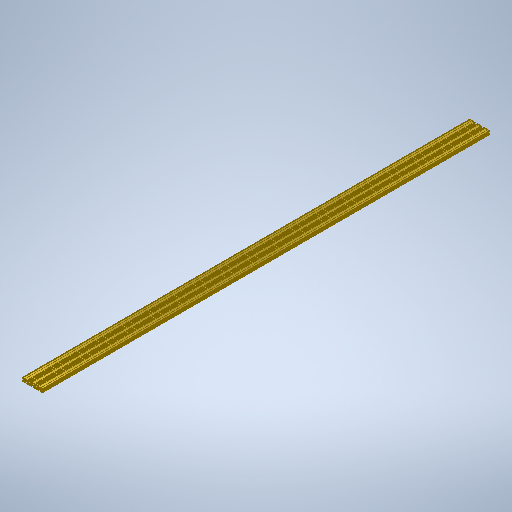
# Autodesk Inventor part: Perfil 15×90 7 rasgos_AST01509007
Saved by Autodesk Inventor 2025.2 (Build 292293000, 293)
## iProperties
Created: 2025-04-03
Part Number: Perfil 15×90 7 rasgos_AST01509007
Material: Ouro
Document SubType Name: Modeling
Designer: Gustavo Sousa
Density: 19.3 g/cm^3
Appearance: Metal quente 2400F
Author: Gustavo Sousa
Autodesk Inventor part; units mm, degrees
ref_plane "YZ Plane" through (0, 0, 0) normal (1, 0, 0) x (0, 1, 0)
ref_plane "XZ Plane" through (0, 0, 0) normal (0, 1, 0) x (-1, 0, 0)
ref_plane "XY Plane" through (0, 0, 0) normal (0, 0, 1) x (1, 0, 0)
sketch "Esboço1" plane through (0, 0, 0) normal (0, 0, 1) x (1, 0, 0)
  line L0 (-45, 7.5) -> (45, 7.5) construction
  line L1 (-45, 7.5) -> (-45, -7.5) construction
  line L2 (-39.5, 3.1) -> (-39.5, -3.1) construction
  line L3 (-45, 3.1) -> (-45, -3.1) construction
  line L4 (-45, 7.5) -> (-45, 3.1) construction
  line L5 (-45, 3.1) -> (-43.5, 3.1) construction
  line L6 (-43.5, 3.1) -> (-43.5, 6.1) construction
  line L7 (-43.5, 6.1) -> (-39.5, 3.1) construction
  line L8 (-45, -3.1) -> (-45, -7.5) construction
  line L9 (-45, -3.1) -> (-43.5, -3.1) construction
  line L10 (-43.5, -3.1) -> (-43.5, -6.1) construction
  line L11 (-43.5, -6.1) -> (-39.5, -3.1) construction
  line L12 (-45, -7.5) -> (45, -7.5) construction
  arc A0 (-44.5, 7.5) -> (-45, 7) centre (-44.5, 7) ccw
  line L13 (-45, 7) -> (-45, 3.1) construction
  line L14 (-34.1, -7.5) -> (-25.9, -7.5) construction
  line L15 (-19.1, 7.5) -> (-10.9, 7.5) construction
  line L16 (-34.1, -7.5) -> (-34.1, -5.3) construction
  line L17 (-25.9, -5.3) -> (-25.9, -7.5) construction
  line L18 (-19.1, 7.5) -> (-19.1, 5.3) construction
  line L19 (-10.9, 7.5) -> (-10.9, 5.3) construction
  line L20 (-25.9, -5.3) -> (-22.7, -5.3) construction
  line L21 (-34.1, -5.3) -> (-37.3, -5.3) construction
  line L22 (-34.1, 0.3735) -> (-25.9, 0.3735) construction
  line L23 (-19.1, -0.3735) -> (-10.9, -0.3735) construction
  line L24 (-25.9, 0.3735) -> (-22.7, -1.1206) construction
  line L25 (-22.3, 1.1206) -> (-19.1, -0.3735) construction
  line L26 (-22.7, -1.1206) -> (-22.7, -5.3) construction
  line L27 (-37.3, -1.1206) -> (-37.3, -5.3) construction
  line L28 (-37.3, -1.1206) -> (-34.1, 0.3735) construction
  line L29 (-19.1, 5.3) -> (-22.3, 5.3) construction
  line L30 (-22.3, 5.3) -> (-22.3, 1.1206) construction
  line L31 (-10.9, 5.3) -> (-7.7, 5.3) construction
  line L32 (-7.7, 5.3) -> (-7.7, 1.1206) construction
  line L33 (-7.7, 1.1206) -> (-10.9, -0.3735) construction
  line L34 (-45, 3.1) -> (-44.5, 3.1) construction
  line L35 (-44.5, 3.1) -> (-44.5, 3.6)
  line L36 (-44.5, 3.6) -> (-45, 3.6)
  line L37 (-45, 3.6) -> (-45, 3.1) construction
  line L38 (-45, 7) -> (-45, 3.6)
  line L39 (-44.5, 3.1) -> (-43.5, 3.1)
  arc A1 (-39.5, 2.85) -> (-39.7, 3.25) centre (-40, 2.85) ccw
  arc A2 (-42.7, 5.5) -> (-43.5, 5.1) centre (-43, 5.1) ccw
  arc A3 (-39.7, -3.25) -> (-39.5, -2.85) centre (-40, -2.85) ccw
  arc A4 (-43.5, -5.1) -> (-42.7, -5.5) centre (-43, -5.1) ccw
  line L40 (-43.5, 5.1) -> (-43.5, 3.1)
  line L41 (-42.7, 5.5) -> (-39.7, 3.25)
  line L42 (-39.5, 2.85) -> (-39.5, -2.85)
  line L43 (-42.7, -5.5) -> (-39.7, -3.25)
  line L44 (-43.5, -5.1) -> (-43.5, -3.1)
  line L45 (-45, -3.1) -> (-44.5, -3.1) construction
  line L46 (-44.5, -3.1) -> (-44.5, -3.6)
  line L47 (-44.5, -3.6) -> (-45, -3.6)
  line L48 (-45, -3.6) -> (-45, -3.1) construction
  line L49 (-44.5, -3.1) -> (-43.5, -3.1)
  arc A5 (-45, -7) -> (-44.5, -7.5) centre (-44.5, -7) ccw
  line L50 (-45, -3.6) -> (-45, -7)
  line L51 (-34.1, -7.5) -> (-34.6, -7.5) construction
  line L52 (-34.6, -7.5) -> (-34.6, -7)
  line L53 (-34.6, -7) -> (-34.1, -7)
  line L54 (-34.1, -7) -> (-34.1, -7.5) construction
  line L55 (-44.5, -7.5) -> (-34.6, -7.5)
  line L56 (-34.1, -7) -> (-34.1, -5.3)
  arc A6 (-37.3, -4.8) -> (-36.8, -5.3) centre (-36.8, -4.8) ccw
  arc A7 (-37.0115, -0.9859) -> (-37.3, -1.439) centre (-36.8, -1.439) ccw
  arc A8 (-33.989, 0.3735) -> (-34.2006, 0.3266) centre (-33.989, -0.1265) ccw
  arc A9 (-25.7994, 0.3266) -> (-26.011, 0.3735) centre (-26.011, -0.1265) ccw
  arc A10 (-22.7, -1.439) -> (-22.9885, -0.9859) centre (-23.2, -1.439) ccw
  arc A11 (-23.2, -5.3) -> (-22.7, -4.8) centre (-23.2, -4.8) ccw
  line L57 (-34.1, -5.3) -> (-36.8, -5.3)
  line L58 (-37.3, -4.8) -> (-37.3, -1.439)
  line L59 (-37.0115, -0.9859) -> (-34.2006, 0.3266)
  line L60 (-33.989, 0.3735) -> (-26.011, 0.3735)
  line L61 (-25.7994, 0.3266) -> (-22.9885, -0.9859)
  line L62 (-22.7, -1.439) -> (-22.7, -4.8)
  line L63 (-23.2, -5.3) -> (-25.9, -5.3)
  line L64 (-25.9, -7.5) -> (-25.4, -7.5) construction
  line L65 (-25.4, -7.5) -> (-25.4, -7)
  line L66 (-25.4, -7) -> (-25.9, -7)
  line L67 (-25.9, -7) -> (-25.9, -7.5) construction
  line L68 (-25.9, -5.3) -> (-25.9, -7)
  line L69 (-4.1, -7.5) -> (4.1, -7.5) construction
  line L70 (-4.1, -5.3) -> (-4.1, -7.5) construction
  line L71 (-7.3, -5.3) -> (-4.1, -5.3) construction
  line L72 (-7.3, -5.3) -> (-7.3, -1.1206) construction
  line L73 (-4.1, 0.3735) -> (4.1, 0.3735) construction
  line L74 (-7.3, -1.1206) -> (-4.1, 0.3735) construction
  line L75 (-4.1, -7.5) -> (-4.6, -7.5) construction
  line L76 (-4.6, -7.5) -> (-4.6, -7)
  line L77 (-4.6, -7) -> (-4.1, -7)
  line L78 (-4.1, -7) -> (-4.1, -7.5) construction
  line L79 (-4.1, -5.3) -> (-4.1, -7)
  arc A12 (-7.3, -4.8) -> (-6.8, -5.3) centre (-6.8, -4.8) ccw
  arc A13 (-7.0115, -0.9859) -> (-7.3, -1.439) centre (-6.8, -1.439) ccw
  arc A14 (-3.989, 0.3735) -> (-4.2006, 0.3266) centre (-3.989, -0.1265) ccw
  line L80 (-6.8, -5.3) -> (-4.1, -5.3)
  line L81 (-7.3, -4.8) -> (-7.3, -1.439)
  line L82 (-7.0115, -0.9859) -> (-4.2006, 0.3266)
  line L83 (-3.989, 0.3735) -> (0, 0.3735)
  line L84 (-19.1, 7.5) -> (-19.6, 7.5) construction
  line L85 (-19.6, 7.5) -> (-19.6, 7)
  line L86 (-19.6, 7) -> (-19.1, 7)
  line L87 (-19.1, 7) -> (-19.1, 7.5) construction
  line L88 (-19.1, 7) -> (-19.1, 5.3)
  arc A15 (-21.8, 5.3) -> (-22.3, 4.8) centre (-21.8, 4.8) ccw
  arc A16 (-19.2006, -0.3266) -> (-18.989, -0.3735) centre (-18.989, 0.1265) ccw
  arc A17 (-11.011, -0.3735) -> (-10.7994, -0.3266) centre (-11.011, 0.1265) ccw
  arc A18 (-7.7, 4.8) -> (-8.2, 5.3) centre (-8.2, 4.8) ccw
  line L89 (-19.1, 5.3) -> (-21.8, 5.3)
  arc A19 (-22.3, 1.439) -> (-22.0115, 0.9859) centre (-21.8, 1.439) ccw
  arc A20 (-7.9885, 0.9859) -> (-7.7, 1.439) centre (-8.2, 1.439) ccw
  line L90 (-22.3, 4.8) -> (-22.3, 1.439)
  line L91 (-22.0115, 0.9859) -> (-19.2006, -0.3266)
  line L92 (-18.989, -0.3735) -> (-11.011, -0.3735)
  line L93 (-10.7994, -0.3266) -> (-7.9885, 0.9859)
  line L94 (-7.7, 1.439) -> (-7.7, 4.8)
  line L95 (-8.2, 5.3) -> (-10.9, 5.3)
  line L96 (-10.9, 7.5) -> (-10.4, 7.5) construction
  line L97 (-10.4, 7.5) -> (-10.4, 7)
  line L98 (-10.4, 7) -> (-10.9, 7)
  line L99 (-10.9, 7) -> (-10.9, 7.5) construction
  line L100 (-10.9, 7) -> (-10.9, 5.3)
  line L101 (-10.4, 7.5) -> (0, 7.5)
  line L102 (-5.5, 5.3) -> (5.5, 5.3) construction
  line L103 (5.5, 5.3) -> (5.5, 2.5735) construction
  line L104 (5.5, 2.5735) -> (-5.5, 2.5735) construction
  line L105 (-5.5, 2.5735) -> (-5.5, 5.3) construction
  line L106 (-5.5, 5.3) -> (5.5, 2.5735) construction
  line L107 (5.5, 5.3) -> (-5.5, 2.5735) construction
  arc A21 (-5, 5.3) -> (-5.5, 4.8) centre (-5, 4.8) ccw
  arc A22 (-5.5, 3.0735) -> (-5, 2.5735) centre (-5, 3.0735) ccw
  arc A23 (5, 2.5735) -> (5.5, 3.0735) centre (5, 3.0735) ccw construction
  arc A24 (5.5, 4.8) -> (5, 5.3) centre (5, 4.8) ccw construction
  line L108 (-5, 5.3) -> (5, 5.3) construction
  line L109 (5.5, 4.8) -> (5.5, 3.0735) construction
  line L110 (-5, 2.5735) -> (5, 2.5735) construction
  line L111 (-5.5, 4.8) -> (-5.5, 3.0735)
  line L112 (-5, 5.3) -> (0, 5.3)
  line L113 (-5, 2.5735) -> (0, 2.5735)
  line L114 (-4.6, -7.5) -> (-25.4, -7.5)
  line L115 (0, 0.3735) -> (0, 2.5735)
  line L116 (0, 7.5) -> (0, 5.3)
  line L117 (-20.5, -2.5735) -> (-9.5, -2.5735) construction
  line L118 (-9.5, -2.5735) -> (-9.5, -5.3) construction
  line L119 (-9.5, -5.3) -> (-20.5, -5.3) construction
  line L120 (-20.5, -5.3) -> (-20.5, -2.5735) construction
  line L121 (-20.5, -2.5735) -> (-9.5, -5.3) construction
  line L122 (-9.5, -2.5735) -> (-20.5, -5.3) construction
  arc A25 (-20, -2.5735) -> (-20.5, -3.0735) centre (-20, -3.0735) ccw
  arc A26 (-20.5, -4.8) -> (-20, -5.3) centre (-20, -4.8) ccw
  arc A27 (-10, -5.3) -> (-9.5, -4.8) centre (-10, -4.8) ccw
  arc A28 (-9.5, -3.0735) -> (-10, -2.5735) centre (-10, -3.0735) ccw
  line L123 (-20, -2.5735) -> (-10, -2.5735)
  line L124 (-20.5, -3.0735) -> (-20.5, -4.8)
  line L125 (-20, -5.3) -> (-10, -5.3)
  line L126 (-9.5, -4.8) -> (-9.5, -3.0735)
  line L127 (-35.5, 5.3) -> (-24.5, 5.3) construction
  line L128 (-24.5, 5.3) -> (-24.5, 2.5735) construction
  line L129 (-24.5, 2.5735) -> (-35.5, 2.5735) construction
  line L130 (-35.5, 2.5735) -> (-35.5, 5.3) construction
  line L131 (-35.5, 5.3) -> (-24.5, 2.5735) construction
  line L132 (-24.5, 5.3) -> (-35.5, 2.5735) construction
  arc A29 (-35, 5.3) -> (-35.5, 4.8) centre (-35, 4.8) ccw
  arc A30 (-35.5, 3.0735) -> (-35, 2.5735) centre (-35, 3.0735) ccw
  arc A31 (-24.5, 4.8) -> (-25, 5.3) centre (-25, 4.8) ccw
  arc A32 (-25, 2.5735) -> (-24.5, 3.0735) centre (-25, 3.0735) ccw
  line L133 (-35, 5.3) -> (-25, 5.3)
  line L134 (-24.5, 4.8) -> (-24.5, 3.0735)
  line L135 (-25, 2.5735) -> (-35, 2.5735)
  line L136 (-35.5, 3.0735) -> (-35.5, 4.8)
  line L137 (-44.5, 7.5) -> (-19.6, 7.5)
  line L138 (0, 0.3735) -> (0, 0)
  point P0 (-45, 0)
  point P1 (-39.5, 0)
  point P2 (-45, 0)
  point P3 (-30, -7.5)
  point P4 (-15, 7.5)
  point P5 (-30, 0.3735)
  point P6 (-15, -0.3735)
  point P7 (-20.7, 0.3735)
  point P8 (-1.9945, 0.3735)
  point P9 (-15, -3.9368)
  point P10 (-15, -0.3735)
  point P11 (-15, -5.3)
  point P12 (-30, 3.9368)
  point P13 (-30, 0.3735)
  point P14 (-30, 5.3)
  dimension "d0" = 90
  dimension "d5" = 15
  dimension "d6" = 5.5
  dimension "d7" = 6.2
  dimension "d9" = 1.5
  dimension "d10" = 3
  dimension "d24" = 0.5
  dimension "d74" = 8.2
  dimension "d75" = 30
  dimension "d76" = 15
  dimension "d79" = 2.2
  dimension "d81" = 2.2
  dimension "d86" = 0.5
  dimension "d87" = 2.2
  dimension "d88" = 2.2
  dimension "espessura" = 2.2
  dimension "d93" = 2.2
  constraints: 278 end point, 70 tangent, 68 point on line, 66 point on circle, 39 equal length, 34 collinear, 33 centre point, 32 equal radius, 30 horizontal, 22 parallel, 21 midpoint, 20 vertical, 12 perpendicular, 6 horizontal alignment, 5 vertical alignment, 2 coincident
  measures "d0" distance of L0.start L0.end
  measures "d5" distance of L0.start L1.end
  measures "d6" distance between parallel lines of L1 L2
  measures "d7" distance of L2.start L2.end
  measures "d9" distance between parallel lines of L1 L6
  measures "d10" distance of L6.end L5.end
  measures "d24" radius of A0
  measures "d74" distance of L14.start L14.end
  measures "d75" horizontal distance of L138.end point (-30, -7.5)
  measures "d76" horizontal distance of L138.end point (-15, 7.5)
  measures "d79" distance between parallel lines of L12 L21
  measures "d81" distance between parallel lines of L25 L24
  measures "d86" distance of L35.end L36.end
  measures "d87" distance from line of point (-1.995, 0.374) L104
  measures "d88" distance between parallel lines of L32 L105
  measures "espessura" distance between parallel lines of L42 L58
  measures "d93" distance between parallel lines of L126 L81
extrude "Extrusão1" add sketch "Esboço1" along normal mid plane 2000
mirror "Espelhar1" about plane through (0, 0, 0) normal (1, 0, 0) of "Extrusão1"
